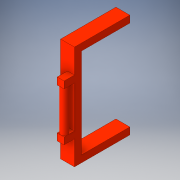
# Autodesk Inventor part: hand
Saved by Autodesk Inventor 2016 (Build 200138000, 138)
## iProperties
Created: 2018-01-19
Part Number: hand
Material: Generic
Document SubType Name: Modeling
Designer: New User
Density: 1 g/cm^3
Appearance: Default
Author: New User
Autodesk Inventor part; units mm, degrees
ref_plane "YZ Plane" through (0, 0, 0) normal (1, 0, 0) x (0, 1, 0)
ref_plane "XZ Plane" through (0, 0, 0) normal (0, 1, 0) x (-1, 0, 0)
ref_plane "XY Plane" through (0, 0, 0) normal (0, 0, 1) x (1, 0, 0)
sketch "Sketch1" plane through (0, 0, 0) normal (0, 1, 0) x (-1, 0, 0)
  line L0 (0, 0) -> (50.8, 0)
  line L1 (50.8, 0) -> (50.8, -203.2)
  line L2 (50.8, -203.2) -> (0, -203.2)
  line L3 (0, -203.2) -> (0, 0)
  dimension "d0" = 50.8
  dimension "d1" = 203.2
  constraints: 8 end point, 2 parallel, 1 horizontal, 1 perpendicular
  measures "d0" distance of L1.end L2.end
  measures "d1" distance of L2.end L0.start
extrude "Extrusion1" add sketch "Sketch1" along normal blind 25.4
sketch "Sketch2" plane through (0, 25.4, 0) normal (0, 1, 0) x (1, 0, 0)
  line L0 (-50.8, 0) -> (0, 0) projected
  line L1 (0, 0) -> (0, 203.2) projected
  line L2 (-50.8, 0) -> (0, 0)
  line L3 (0, 0) -> (0, 25.4)
  line L4 (0, 25.4) -> (-50.8, 25.4)
  line L5 (-50.8, 25.4) -> (-50.8, 0)
  dimension "d4" = 25.4
  constraints: 8 end point, 2 parallel, 1 horizontal, 1 perpendicular, 1 point on line
  measures "d4" distance of L4.end L0.start
extrude "Extrusion2" add sketch "Sketch2" along normal blind 330.2
sketch "Sketch3" plane through (0, 355.6, 0) normal (0, 1, 0) x (1, 0, 0)
  line L0 (0, 203.2) -> (-50.8, 203.2) projected
  line L1 (0, 0) -> (-50.8, 0)
  line L2 (-50.8, 0) -> (-50.8, 203.2)
  line L3 (-50.8, 203.2) -> (0, 203.2)
  line L4 (0, 203.2) -> (0, 0)
  constraints: 8 end point, 2 parallel, 1 horizontal, 1 perpendicular
extrude "Extrusion3" add sketch "Sketch3" along normal blind 25.4
sketch "Sketch4" plane through (-50.8, 0, 0) normal (0, 0, 1) x (1, 0, 0)
  line L0 (50.8, 292.1) -> (25.4, 292.1)
  line L1 (25.4, 292.1) -> (25.4, 266.7)
  line L2 (25.4, 266.7) -> (50.8, 266.7)
  line L3 (50.8, 266.7) -> (50.8, 292.1)
  line L4 (50.8, 88.9) -> (25.4, 88.9)
  line L5 (25.4, 88.9) -> (25.4, 114.3)
  line L6 (25.4, 114.3) -> (50.8, 114.3)
  line L7 (50.8, 114.3) -> (50.8, 88.9)
  line L8 (50.8, 0) -> (0, 0) projected
  dimension "d19" = 152.4
  dimension "d20" = 25.4
  dimension "d21" = 25.4
  dimension "d22" = 88.9
  constraints: 16 end point, 4 parallel, 2 horizontal, 2 perpendicular, 1 collinear, 1 point on line
  measures "d19" distance between parallel lines of L6 L2
  measures "d20" distance of L1.end L2.end
  measures "d21" distance of L4.end L5.end
  measures "d22" distance between parallel lines of L8 L4
extrude "Extrusion4" add sketch "Sketch4" along normal blind 38.1
sketch "Sketch6" plane through (-25.4, 114.3, 0) normal (0, 1, 0) x (1, 0, 0)
  circle A0 centre (12.7, -25.4) radius 12.7
  line L0 (25.4, 0) -> (25.4, -38.1) projected
  line L1 (25.4, -38.1) -> (0, -38.1) projected
  dimension "d23" = 25.4
  dimension "d24" = 12.7
  dimension "d25" = 12.7
  constraints: 1 centre point
  measures "d23" diameter of A0
  measures "d24" distance from line of L0 A0.centre
  measures "d25" distance from line of L1 A0.centre
extrude "Extrusion5" add sketch "Sketch6" along normal blind 158.75 contours A0
body "Solid1"
